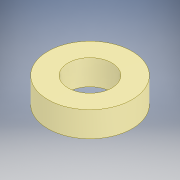
# Autodesk Inventor part: HPW-5.2-10-3-N
Saved by Autodesk Inventor 2019 (Build 230136000, 136)
## iProperties
Created: 2018-05-06
Part Number: HPW-5.2-10-3-N
Material: Nylon 6/6
Document SubType Name: Modeling
Designer: IEUser
Density: 1.13 g/cm^3
Appearance: Nylon 6
Author: IEUser
Autodesk Inventor part; units mm, degrees
ref_plane "YZ Plane" through (0, 0, 0) normal (1, 0, 0) x (0, 1, 0)
ref_plane "XZ Plane" through (0, 0, 0) normal (0, 1, 0) x (-1, 0, 0)
ref_plane "XY Plane" through (0, 0, 0) normal (0, 0, 1) x (1, 0, 0)
sketch "Washer Cross Section" plane through (0, 0, 0) normal (0, 1, 0) x (-1, 0, 0)
  circle A0 centre (0, 0) radius 5
  circle A1 centre (0, 0) radius 2.6
  dimension "d0" = 10
  dimension "d1" = 5.2
  constraints: 2 centre point, 2 coincident
  measures "d0" diameter of A0
  measures "d1" diameter of A1
extrude "Washer" add sketch "Washer Cross Section" along normal blind 3
body "Solid1"
